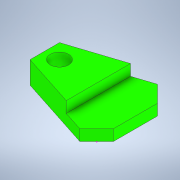
# Autodesk Inventor part: rollertriangle(v3)
Saved by Autodesk Inventor 2022 (Build 260153000, 153)
## iProperties
Created: 2022-11-07
Part Number: rollertriangle(v3)
Material: Generic
Document SubType Name: Modeling
Designer: matia
Density: 1 g/cm^3
Appearance: Default
Author: matia
Autodesk Inventor part; units mm, degrees
ref_plane "YZ Plane" through (0, 0, 0) normal (1, 0, 0) x (0, 1, 0)
ref_plane "XZ Plane" through (0, 0, 0) normal (0, 1, 0) x (-1, 0, 0)
sketch "Sketch1" plane through (0, 0, 0) normal (0, 1, 0) x (-1, 0, 0)
  circle A0 centre (0, 0) radius 1.5875
  line L0 (0, 0) -> (0, -7.62)
  circle A1 centre (0, -7.62) radius 1.5875
  line L1 (-14.0081, -3.81) -> (-6.6675, -3.81)
  circle A2 centre (10.1981, -3.81) radius 1.5875
  line L2 (10.1981, -3.81) -> (10.1981, -6.35)
  line L3 (10.1981, -6.35) -> (10.1981, -1.27)
  line L4 (0, 1.5875) -> (0, 2.8575)
  line L5 (-1.5875, 0) -> (-2.8575, 0)
  line L6 (0, -9.2075) -> (0, -10.4775)
  line L7 (-1.5875, -7.62) -> (-2.8575, -7.62)
  line L8 (-2.8575, -7.62) -> (-2.8575, 0)
  line L9 (0, 2.8575) -> (-2.8575, 0)
  line L10 (0, 2.8575) -> (3.4925, 1.444)
  line L11 (3.4925, -9.064) -> (0, -10.4775)
  line L12 (-2.8575, -7.62) -> (0, -10.4775)
  line L13 (-2.8575, -3.81) -> (0, -3.81)
  line L14 (3.4925, -3.81) -> (3.4925, -9.064)
  line L15 (3.4925, -3.81) -> (3.4925, 1.444)
  line L16 (10.1981, -3.81) -> (12.7381, -3.81)
  line L17 (12.7381, -3.81) -> (12.7381, -6.35)
  line L18 (12.7381, -6.35) -> (10.1981, -6.35)
  line L19 (12.7381, -3.81) -> (12.7381, -1.27)
  line L20 (12.7381, -1.27) -> (10.1981, -1.27)
  line L21 (12.7381, -6.35) -> (0, -10.4775)
  line L22 (12.7381, -1.27) -> (0, 2.8575)
  line L23 (10.1981, -3.81) -> (12.7381, -3.81)
  line L24 (3.4925, 1.444) -> (3.4925, 1.7258)
  line L25 (3.4925, -9.064) -> (3.4925, -9.3458)
  dimension "d0" = 3.175
  dimension "d1" = 7.62
  dimension "d2" = 3.175
  dimension "d3" = 7.3406
  dimension "d4" = 3.175
  dimension "d7" = 5.08
  dimension "d8" = 1.27
  dimension "d9" = 1.27
  dimension "d10" = 1.27
  dimension "d11" = 1.27
  dimension "d12" = 6.35
  dimension "d44" = 2.54
  constraints: 52 end point, 7 point on line, 6 perpendicular, 5 horizontal, 4 point on circle, 4 vertical, 3 centre point, 2 coincident, 2 midpoint, 1 collinear
  measures "d0" diameter of A0
  measures "d1" distance of L0.start L0.end
  measures "d2" diameter of A1
  measures "d3" distance of L1.start L1.end
  measures "d4" diameter of A2
  measures "d7" distance of L2.end L3.end
  measures "d8" distance of L4.start L4.end
  measures "d9" distance of L5.start L5.end
  measures "d10" distance of L6.start L6.end
  measures "d11" distance of L7.start L7.end
  measures "d12" distance of L13.start L14.start
  measures "d44" distance of L16.end L23.start
ref_plane "Work Plane2" through (2.8575, 0, 0) normal (0.7071, 0, 0.7071) x (0.7071, 0, -0.7071)
sketch "Sketch3" plane through (2.8575, 0, 0) normal (0.7071, 0, 0.7071) x (0.7071, 0, -0.7071)
  point P0 (-2.0206, 0)
extrude "Extrusion4" add sketch "Sketch1" along normal blind 1.905 contours A0 L4 L10 L15 L14 L11 L6 A1 L0 | A0 L5 L9 L4 | L0 L13 L8 L5 A0 | L22 L24 L10 | L0 A1 L7 L8 L13 | A1 L6 L12 L7 | L25 L21 L11
extrude "Extrusion5" add sketch "Sketch1" along normal blind 3.81 contours L24 L22 L20 L3 A2 L2 L18 L21 L25 L14 L15 | L19 L16 A2 L3 L20 | L17 L18 L2 A2 L16
extrude "Extrusion6" add sketch "Sketch1" along normal blind 1.905 contours A0 | A1
body "Solid2"
